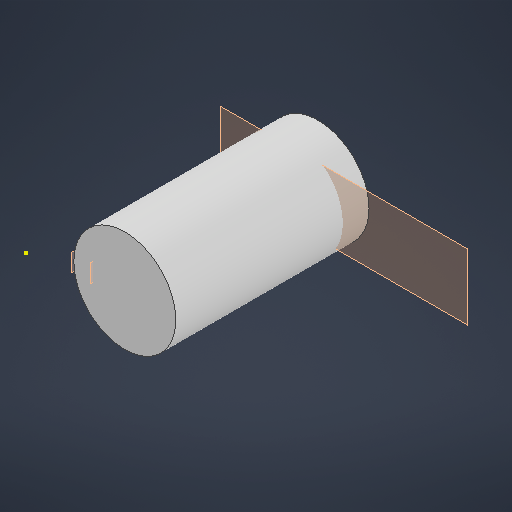
# Autodesk Inventor part: rim-v1
Saved by Autodesk Inventor 2026.2 (Build 302298010, 298A)
## iProperties
Created: 2026-05-11
Part Number: rim-v1
Material: Generic
Document SubType Name: Modeling
Designer: karol
Density: 1 g/cm^3
Appearance: Default
Author: karol
Autodesk Inventor part; units mm, degrees
ref_plane "YZ Plane" through (0, 0, 0) normal (1, 0, 0) x (0, 1, 0)
ref_plane "XZ Plane" through (0, 0, 0) normal (0, 1, 0) x (-1, 0, 0)
ref_plane "XY Plane" through (0, 0, 0) normal (0, 0, 1) x (1, 0, 0)
ref_plane "Work Plane1" through (0, 0, 0.5) normal (0, 0, 1) x (1, 0, 0)
sketch "Sketch1" plane through (0, 0, 0.5) normal (0, 0, 1) x (1, 0, 0)
  arc A0 (13, 1.882) -> (13, 4.118) centre (14, 3) ccw projected
  arc A1 (13, 1.882) -> (13, 4.118) centre (14, 3) ccw projected
  line L0 (13, 4.118) -> (13, 1.882) projected
  circle A2 centre (14, 3) radius 6
  circle A3 centre (14, 3) radius 4
  circle A4 centre (14, 3) radius 1.7
  line L1 (12.7, 1.9046) -> (12.7, 4.0954)
  point P0 (0, 0)
  dimension "d0" = 12
  dimension "d1" = 8
  dimension "d2" = 0.2
  dimension "d3" = 0.3
  constraints: 3 centre point, 3 coincident, 2 end point, 2 point on circle, 1 parallel, 1 vertical
  measures "d0" diameter of A2
  measures "d1" diameter of A3
  measures "d2" radial gap between concentric circles of A0 A4
  measures "d3" distance between parallel lines of L0 L1
extrude "Extrusion1" add sketch "Sketch1" along normal blind 21.5 contours A3 | L1 A4 picked at (12.5667, 3)
ref_plane "Work Plane2" through (14, 3, 18) normal (0, 0, 1) x (1, 0, 0)
sketch "Sketch2" plane through (14, 3, 18) normal (0, 0, 1) x (1, 0, 0)
  circle A0 centre (0, 0) radius 4 projected
  arc A1 (-1.3, -1.0954) -> (-1.3, 1.0954) centre (0, 0) ccw projected
  line L0 (-1.3, -1.0954) -> (-1.3, 1.0954) projected
  circle A2 centre (0, 0) radius 3
  point P0 (-14, -3)
  dimension "d7" = 6
  constraints: 1 centre point, 1 coincident
  measures "d7" diameter of A2
extrude "Extrusion2" cut sketch "Sketch2" against normal blind 2 contours A0
ref_plane "Work Plane3" through (9.7, 1.9046, 0.5) normal (1, 0, 0) x (0, 0, -1)
sketch "Sketch3" plane through (9.7, 1.9046, 0.5) normal (1, 0, 0) x (0, 0, -1)
  circle A0 centre (-2.5, 1) radius 1.42
  line L0 (-21.5, 0) -> (-21.5, 2.1909) projected
  point P0 (0.5, -1.9046)
  dimension "d11" = 2.84
  dimension "d12" = 1
  dimension "d15" = 19
  constraints: 1 centre point
  measures "d11" diameter of A0
  measures "d12" vertical distance of L0.start A0.centre
  measures "d15" distance from line of L0 A0.centre
extrude "Extrusion3" cut sketch "Sketch3" along normal blind 3
chamfer "Chamfer1" distance 0.25 angle 45 1 edges at (10.0014, 2.8952, 4.42)
ref_plane "Work Plane4" through (14, 3, 13) normal (0, 0, 1) x (1, 0, 0)
sketch "Sketch4" plane through (14, 3, 13) normal (0, 0, 1) x (1, 0, 0)
  circle A0 centre (0, 0) radius 4 projected
  circle A1 centre (0, 0) radius 4 projected
  circle A2 centre (0, 0) radius 3 projected
  point P0 (-14, -3)
extrude "Extrusion4" cut sketch "Sketch4" against normal blind 2
sketch "Sketch5" plane through (14, 3, 22) normal (0, 0, 1) x (1, 0, 0)
  point P0 (-14, -3)
sketch "Sketch6" plane through (14, 3, 22) normal (0, 0, 1) x (1, 0, 0)
  circle A0 centre (0, 0) radius 3 projected
  circle A1 centre (0, 0) radius 6
  circle A2 centre (0, 0) radius 6.8
  point P0 (-14, -3)
  dimension "d22" = 12
  dimension "d23" = 13.6
  constraints: 2 centre point, 2 coincident
  measures "d22" diameter of A1
  measures "d23" diameter of A2
extrude "Extrusion8" add sketch "Sketch6" against normal blind 25 contours A2
extrude "Extrusion9" add sketch "Sketch6" along normal blind 0.8 contours A0 | A1 | A2
ref_plane "Work Plane6" through (7.2, 1.9046, 0.5) normal (1, 0, 0) x (0, 0, -1)
sketch "Sketch8" plane through (7.2, 1.9046, 0.5) normal (1, 0, 0) x (0, 0, -1)
  circle A0 centre (-2.5, 1) radius 1.5
  arc A1 (-1.4918, 0) -> (-1.7266, 2.1909) centre (-2.5, 1) ccw projected
  point P0 (0.5, -1.9046)
  dimension "d36" = 3
  constraints: 1 centre point, 1 concentric, 1 other
  measures "d36" diameter of A0
extrude "Extrusion10" cut sketch "Sketch8" along normal blind 2
body "Solid1"
